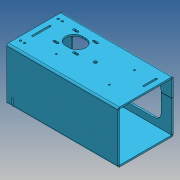
# Autodesk Inventor part: exquema
Saved by Autodesk Inventor 2017 (Build 210142000, 142)
## iProperties
Part Number: exquema
Material: Genérico
Document SubType Name: Chapa
Designer: Leo
Density: 1 g/cm^3
Appearance: Turquesa
Sheet Metal Rule: Por defecto
Flat Pattern Width: 53.096 cm
Flat Pattern Length: 26.5 cm
Flat Pattern Area: 1407.04 cm^2
Sheet Metal Width: 530,960 mm
Sheet Metal Length: 265,000 mm
Sheet Metal Area: 140704,415 mm^2
Author: Leo
Autodesk Inventor part; units mm, degrees
ref_plane "YZ Plane" through (0, 0, 0) normal (1, 0, 0) x (0, 1, 0)
ref_plane "XZ Plane" through (0, 0, 0) normal (0, 1, 0) x (-1, 0, 0)
ref_plane "XY Plane" through (0, 0, 0) normal (0, 0, 1) x (1, 0, 0)
sketch "Boceto1" plane through (0, 0, 0) normal (0, 0, 1) x (1, 0, 0)
  circle A0 centre (0, 0) radius 3.175
  circle A1 centre (0, 0) radius 10 construction
  circle A2 centre (65.0377, -18.065) radius 57.5 construction
  line L0 (28.2, 28.2) -> (-28.2, 28.2) construction
  line L1 (-28.2, 28.2) -> (-28.2, -28.2) construction
  line L2 (-28.2, -28.2) -> (28.2, -28.2) construction
  line L3 (28.2, -28.2) -> (28.2, 28.2) construction
  line L4 (-4.8788, 8.7291) -> (36.9844, 32.1272) construction
  line L5 (15.1172, -46.599) -> (-8.6818, -4.9624) construction
  line L6 (-28.2, -36.2) -> (171.8, -36.2) construction
  line L7 (171.8, -36.2) -> (171.8, -78.2) construction
  line L8 (171.8, -78.2) -> (-28.2, -78.2) construction
  line L9 (-28.2, -78.2) -> (-28.2, -36.2) construction
  circle A3 centre (65.0377, -18.065) radius 4
  line L10 (-19.57, 21.07) -> (-27.57, 21.07)
  arc A4 (-27.57, 26.07) -> (-27.57, 21.07) centre (-27.57, 23.57) ccw
  line L11 (-27.57, 26.07) -> (-19.57, 26.07)
  arc A5 (-19.57, 21.07) -> (-19.57, 26.07) centre (-19.57, 23.57) ccw
  line L12 (19.57, -21.07) -> (27.57, -21.07)
  arc A6 (27.57, -26.07) -> (27.57, -21.07) centre (27.57, -23.57) ccw
  line L13 (27.57, -26.07) -> (19.57, -26.07)
  arc A7 (19.57, -21.07) -> (19.57, -26.07) centre (19.57, -23.57) ccw
  line L14 (19.57, 26.07) -> (27.57, 26.07)
  arc A8 (27.57, 21.07) -> (27.57, 26.07) centre (27.57, 23.57) ccw
  line L15 (27.57, 21.07) -> (19.57, 21.07)
  arc A9 (19.57, 26.07) -> (19.57, 21.07) centre (19.57, 23.57) ccw
  line L16 (-19.57, 23.57) -> (-27.57, 23.57) construction
  line L17 (19.57, 23.57) -> (27.57, 23.57) construction
  line L18 (48.6318, -18.065) -> (81.4437, -18.065) construction
  circle A10 centre (128.2833, 11.935) radius 2
  circle A11 centre (128.2833, -48.065) radius 2
  circle A12 centre (128.2833, 11.935) radius 12.5 construction
  circle A13 centre (65.0377, -18.065) radius 30 construction
  line L19 (125.683, -0.2916) -> (71.2783, 11.2787) construction
  line L20 (-78.2, 46.07) -> (186.8, 46.07)
  line L21 (186.8, 46.07) -> (186.8, -82.2)
  line L22 (186.8, -82.2) -> (-78.2, -82.2)
  line L23 (-78.2, -82.2) -> (-78.2, 46.07)
  circle A14 centre (1.7922, -48.065) radius 2
  circle A15 centre (1.7922, -48.065) radius 12.5 construction
  circle A16 centre (65.0377, -18.065) radius 11 construction
  line L24 (-27.57, -21.07) -> (-19.57, -21.07)
  arc A17 (-19.57, -26.07) -> (-19.57, -21.07) centre (-19.57, -23.57) ccw
  line L25 (-19.57, -26.07) -> (-27.57, -26.07)
  arc A18 (-27.57, -21.07) -> (-27.57, -26.07) centre (-27.57, -23.57) ccw
  line L26 (-27.57, -23.57) -> (-19.57, -23.57) construction
  line L27 (-23.57, -23.57) -> (-23.57, 23.57) construction
  line L28 (23.57, 23.57) -> (23.57, -18.9602) construction
  line L29 (-23.57, 0) -> (23.57, 0) construction
  line L30 (-4, -20) -> (4, -20)
  arc A19 (4, -20) -> (4, 20) centre (4, 0) ccw
  line L31 (4, 20) -> (-4, 20)
  arc A20 (-4, 20) -> (-4, -20) centre (-4, 0) ccw
  line L32 (-65.7, 2.435) -> (-65.7, -38.565)
  arc A21 (-65.7, -38.565) -> (-61.7, -38.565) centre (-63.7, -38.565) ccw
  line L33 (-61.7, -38.565) -> (-61.7, 2.435)
  arc A22 (-61.7, 2.435) -> (-65.7, 2.435) centre (-63.7, 2.435) ccw
  circle A23 centre (-68.7, -63.065) radius 2.5
  circle A24 centre (-58.7, -63.065) radius 2.5
  line L34 (-68.7, -63.065) -> (-58.7, -63.065) construction
  circle A25 centre (-68.7, 26.935) radius 2.5
  circle A26 centre (-58.7, 26.935) radius 2.5
  line L35 (174.3, 20) -> (174.3, -9.3223)
  arc A27 (170.3, -9.3223) -> (174.3, -9.3223) centre (172.3, -9.3223) ccw
  line L36 (170.3, -9.3223) -> (170.3, 20)
  arc A28 (174.3, 20) -> (170.3, 20) centre (172.3, 20) ccw
  point P0 (-28.2, 0)
  point P1 (0, -28.2)
  point P2 (54.3, -82.2)
  point P3 (186.8, -18.065)
  point P4 (0, 20)
  point P5 (-65.7, -18.065)
  point P6 (-78.2, -18.065)
  point P7 (-63.7, -63.065)
  dimension "d15" = 25
  dimension "d17" = 60
  dimension "d0" = 6.35
  dimension "d1" = 56.4
  dimension "d2" = 67.5
  dimension "d4" = 200
  dimension "d5" = 42
  dimension "d6" = 8
  dimension "d7" = 11.235
  dimension "d8" = 5
  dimension "d9" = 39.14
  dimension "d10" = 8
  dimension "d11" = 55.14
  dimension "d12" = 8
  dimension "d13" = 4
  dimension "d14" = 115
  dimension "d16" = 60
  dimension "d18" = 4
  dimension "d19" = 20
  dimension "d20" = 22
  dimension "d21" = 128.27
  dimension "d22" = 50
  dimension "d23" = 25
  dimension "d42" = 47.14
  dimension "d43" = 47.14
  dimension "d44" = 20
  dimension "d45" = 8
  dimension "d46" = 8
  dimension "d47" = 15
  dimension "d62" = 4
  dimension "d63" = 41
  dimension "d64" = 12.5
  dimension "d65" = 5
  dimension "d66" = 10
  dimension "d67" = 7
  dimension "d68" = 45
  dimension "d69" = 12.5
  dimension "d70" = 4
  constraints: 75 end point, 34 tangent, 32 point on circle, 27 centre point, 14 midpoint, 14 parallel, 10 horizontal, 9 coincident, 7 horizontal alignment, 7 vertical alignment, 5 equal radius, 5 perpendicular, 3 equal length, 3 point on line, 2 symmetric about line, 2 vertical, 1 collinear, 13 other
  measures "d0" diameter of A0
  measures "d1" distance of L0.end L1.end
  measures "d2" distance of A2.centre point (0, 0)
  measures "d4" distance of L7.end L8.end
  measures "d5" distance of L6.end L7.end
  measures "d6" diameter of A3
  measures "d7" distance edge to line of A2 L0
  measures "d8" distance between parallel lines of L11 L10
  measures "d9" distance of L17.start L16.start
  measures "d10" distance of L16.start L16.end
  measures "d11" distance of L17.end L16.end
  measures "d12" distance of L16.start L16.end
  measures "d13" diameter of A10
  measures "d14" diameter of A2
  measures "d16" distance of point (128.283, 11.935) A11.centre
  measures "d18" distance between parallel lines of L22 L8
  measures "d19" distance edge to line of A4 L20
  measures "d20" diameter of A16
  measures "d21" distance of L20.end L21.end
  measures "d22" distance between parallel lines of L23 L9
  measures "d23" diameter of A15
  measures "d42" distance from line of L26.start L16
  measures "d43" distance between parallel lines of L28 L27
  measures "d44" radius of A20
  measures "d45" distance of L30.start L30.end
  measures "d46" distance between parallel lines of L2 L6
  measures "d47" distance between parallel lines of L21 L7
  measures "d62" distance between parallel lines of L33 L32
  measures "d63" distance of L32.start L32.end
  measures "d64" distance between parallel lines of L23 L32
  measures "d65" diameter of A24
  measures "d66" distance of L34.start L34.end
  measures "d67" distance edge to line of A23 L23
  measures "d68" distance from line of L34 point (-65.7, -18.065)
  measures "d69" distance between parallel lines of L21 L35
  measures "d70" distance between parallel lines of L36 L35
extrude "Extrusión1" add sketch "Boceto1" along normal blind 4 contours L20 L21 L22 L23
sketch "Boceto3" plane through (-68.7083, 50.17, -120) normal (0, 1, 0) x (1, 0, 0)
  line L0 (0, -119.9) -> (265, -119.9) construction
  line L1 (265, 0) -> (265, -119.9) construction
  line L2 (0, 0) -> (265, 0) construction
  line L3 (0, -119.9) -> (0, 0) construction
  line L4 (136.5, -57.95) -> (128.5, -57.95)
  arc A0 (128.5, -57.95) -> (128.5, -61.95) centre (128.5, -59.95) ccw
  line L5 (128.5, -61.95) -> (136.5, -61.95)
  arc A1 (136.5, -61.95) -> (136.5, -57.95) centre (136.5, -59.95) ccw
  line L6 (238, -57.95) -> (230, -57.95)
  arc A2 (230, -57.95) -> (230, -61.95) centre (230, -59.95) ccw
  line L7 (230, -61.95) -> (238, -61.95)
  arc A3 (238, -61.95) -> (238, -57.95) centre (238, -59.95) ccw
  line L8 (35, -57.95) -> (27, -57.95)
  arc A4 (27, -57.95) -> (27, -61.95) centre (27, -59.95) ccw
  line L9 (27, -61.95) -> (35, -61.95)
  arc A5 (35, -61.95) -> (35, -57.95) centre (35, -59.95) ccw
  point P0 (68.7083, -120)
  point P1 (265, -59.95)
  point P2 (132.5, 0)
  point P3 (132.5, -57.95)
  dimension "d36" = 4
  dimension "d37" = 8
  dimension "d38" = 25
  dimension "d39" = 25
  constraints: 12 end point, 12 point on circle, 12 tangent, 6 centre point, 3 horizontal, 3 horizontal alignment, 3 midpoint, 3 parallel, 2 collinear, 2 equal radius, 1 vertical alignment
  measures "d36" distance between parallel lines of L5 L4
  measures "d37" distance of L5.start L5.end
  measures "d38" distance edge to line of A4 L3
  measures "d39" distance edge to line of A3 L1
sketch "Boceto2" plane through (-78.2, -82.3, -0.1) normal (0, -1, 0) x (1, 0, 0)
  line L0 (265, 0) -> (0, 0)
  line L1 (0, 0) -> (0, -119.9)
  line L2 (0, -119.9) -> (265, -119.9)
  line L3 (265, -119.9) -> (265, 0)
  constraints: 6 end point, 1 horizontal, 1 perpendicular, 1 vertical
edge flange "Pestaña1" height 120 angle 90 thickness 4 bend radius 0.1 thickness toward (0, -1, 0) relief tear relief width 4 relief depth 2 edges at (54.3, -82.2, 0) wall of the first edge with corners at (186.8, -82.3, -0.1) (-78.2, -82.3, -0.1) (-78.2, -82.3, -120) (186.8, -82.3, -120)
bend "Doblez1"
corner "Esquina1"
sketch "Boceto4" plane through (-78.2, 46.07, 0) normal (0, 1, 0) x (1, 0, 0)
  line L0 (265, 120) -> (0, 120)
  line L1 (0, 0) -> (265, 0)
  line L2 (0, 120) -> (0, 80.1667)
  line L3 (0, 80.1667) -> (25, 80.1667)
  line L4 (25, 80.1667) -> (25, 83.4303)
  arc A0 (41.5697, 100) -> (25, 83.4303) centre (41.5697, 83.4303) ccw
  line L5 (41.5697, 100) -> (223.4303, 100)
  arc A1 (240, 83.4303) -> (223.4303, 100) centre (223.4303, 83.4303) ccw
  line L6 (240, 83.4303) -> (240, 40.3333)
  line L7 (240, 40.3333) -> (265, 40.3333)
  line L8 (265, 120) -> (265, 40.3333)
  line L9 (265, 0) -> (265, 39.8333)
  line L10 (265, 39.8333) -> (240, 39.8333)
  line L11 (240, 39.8333) -> (240, 36.5697)
  arc A2 (223.4303, 20) -> (240, 36.5697) centre (223.4303, 36.5697) ccw
  line L12 (223.4303, 20) -> (41.5697, 20)
  arc A3 (25, 36.5697) -> (41.5697, 20) centre (41.5697, 36.5697) ccw
  line L13 (25, 36.5697) -> (25, 79.6667)
  line L14 (25, 79.6667) -> (0, 79.6667)
  line L15 (0, 79.6667) -> (0, 0)
  line L16 (254.5, 27.7391) -> (254.5, 68.7391)
  arc A4 (254.5, 68.7391) -> (250.5, 68.7391) centre (252.5, 68.7391) ccw
  line L17 (250.5, 68.7391) -> (250.5, 27.7391)
  arc A5 (250.5, 27.7391) -> (254.5, 27.7391) centre (252.5, 27.7391) ccw
  line L18 (10.5, 51.123) -> (10.5, 92.123)
  arc A6 (14.5, 92.123) -> (10.5, 92.123) centre (12.5, 92.123) ccw
  line L19 (14.5, 92.123) -> (14.5, 51.123)
  arc A7 (10.5, 51.123) -> (14.5, 51.123) centre (12.5, 51.123) ccw
  point P0 (196.907, 99.9603)
  point P1 (265, 0)
  point P2 (265, 120)
  point P3 (0, 120)
  point P4 (252.5, 39.8333)
  point P5 (12.5, 79.6667)
  dimension "d58" = 0.5
  dimension "d59" = 0.5
  dimension "d60" = 20
  dimension "d61" = 20
  dimension "d71" = 25
  dimension "d72" = 25
  dimension "d78" = 4
  dimension "d79" = 41
  dimension "d80" = 39.8333
  dimension "d81" = 79.6667
  constraints: 40 end point, 16 point on circle, 16 tangent, 10 perpendicular, 8 centre point, 6 vertical, 4 coincident, 4 equal radius, 4 parallel, 2 collinear, 2 midpoint, 2 vertical alignment
  measures "d58" distance between parallel lines of L10 L7
  measures "d59" distance between parallel lines of L14 L3
  measures "d60" distance between parallel lines of L1 L12
  measures "d61" distance between parallel lines of L0 L5
  measures "d71" distance between parallel lines of L15 L13
  measures "d72" distance between parallel lines of L8 L6
  measures "d78" distance between parallel lines of L17 L16
  measures "d79" distance of L16.start L16.end
  measures "d80" distance of L1.end L9.end
  measures "d81" distance of L0.start L7.end
sheet face with bend "Cara1" sketch "Boceto4" thickness 4 toward (0, -1, 0) bend radius 0.1 relief tear relief width 4 relief depth 2 contours L8 L7 L16 A4 L17 L6 A1 L5 A0 L4 L3 L19 A6 L18 L2 L0 | L7 L17 A4 L16 | L18 A6 L19 L3
bend "Doblez2"
sheet face with bend "Cara2" sketch "Boceto4" thickness 4 toward (0, -1, 0) bend radius 0.1 relief tear relief width 4 relief depth 2 contours L16 A5 L17 L10 | L10 L9 L1 L15 L14 L18 A7 L19 L13 A3 L12 A2 L11 L17 A5 L16 | L14 L19 A7 L18
bend "Doblez3"
sketch "Boceto5" plane through (186.8, 46.07, -120) normal (0, 0, -1) x (-1, 0, 0)
  line L0 (0, -4) -> (265, -4) projected
  line L1 (0, -128.37) -> (265, -128.37) projected
  line L2 (265, 0) -> (265, -4) projected
  line L3 (265, -4) -> (265, -128.37)
  line L4 (0, -128.37) -> (0, -4)
  line L5 (252.5, -84.635) -> (252.5, -43.635) projected
  arc A0 (252.5, -43.635) -> (248.5, -43.635) centre (250.5, -43.635) ccw projected
  line L6 (248.5, -43.635) -> (248.5, -84.635) projected
  arc A1 (248.5, -84.635) -> (252.5, -84.635) centre (250.5, -84.635) ccw projected
  line L7 (252.5, 1) -> (252.5, -24.185)
  arc A2 (248.5, -24.185) -> (252.5, -24.185) centre (250.5, -24.185) ccw
  line L8 (248.5, -24.185) -> (248.5, 1)
  line L9 (248.5, 1) -> (252.5, 1)
  line L10 (265, -4.1) -> (265, -128.27) projected
  line L11 (265, -66.185) -> (321.347, -66.185)
  line L12 (252.5, -133.37) -> (252.5, -108.185)
  arc A3 (252.5, -108.185) -> (248.5, -108.185) centre (250.5, -108.185) ccw
  line L13 (248.5, -108.185) -> (248.5, -133.37)
  line L14 (248.5, -133.37) -> (252.5, -133.37)
  point P0 (186.8, -46.07)
  dimension "d82" = 84
  dimension "d83" = 5
  constraints: 18 end point, 4 perpendicular, 4 point on circle, 4 tangent, 2 centre point, 2 collinear, 2 parallel, 2 vertical, 1 horizontal, 1 midpoint, 3 other
  measures "d82" distance of A3.centre A2.centre
  measures "d83" distance between parallel lines of L14 L1
sheet face with bend "Cara3" sketch "Boceto5" thickness 4 toward (0, 0, 1) bend radius 0.1 relief tear relief width 4 relief depth 2 contours L0 L8 A2 L7 L3 L1 L12 A3 L13 L4 | L0 L7 A2 L8 | L13 A3 L12 L1 | A1 L6 A0 L5
bend "Doblez4"
extrude "Extrusión3" cut sketch "Boceto5" against normal blind 20 contours L8 L9 L7 L0 | L0 L7 A2 L8 | L13 A3 L12 L1 | L1 L12 L14 L13
